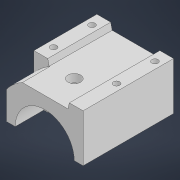
# Autodesk Inventor part: led_holder_01
Saved by Autodesk Inventor 2022 (Build 260153000, 153)
## iProperties
Created: 2025-10-28
Part Number: led_holder_01
Material: 一般
Document SubType Name: Modeling
Designer: gisen
Density: 1 g/cm^3
Appearance: 既定
Author: gisen
Autodesk Inventor part; units mm, degrees
ref_plane "YZ Plane" through (0, 0, 0) normal (1, 0, 0) x (0, 1, 0)
ref_plane "XZ Plane" through (0, 0, 0) normal (0, 1, 0) x (-1, 0, 0)
ref_plane "XY Plane" through (0, 0, 0) normal (0, 0, 1) x (1, 0, 0)
sketch "スケッチ1" plane through (0, 0, 0) normal (0, 0, 1) x (1, 0, 0)
  line L0 (-12.5, 3.2) -> (-11.75, 0)
  line L1 (-11.75, 0) -> (11.75, 0)
  line L2 (11.75, 0) -> (12.5, 3.2)
  line L3 (12.5, 3.2) -> (19.5, 3.2)
  line L4 (19.5, 3.2) -> (19.5, -4)
  line L5 (19.5, -4) -> (-19.5, -4)
  line L6 (-19.5, -4) -> (-19.5, 3.2)
  line L7 (-19.5, 3.2) -> (-12.5, 3.2)
  circle A0 centre (0, -21) radius 12.7 construction
  line L8 (-5.5, -4) -> (5.5, -4) construction
  line L9 (5.5, -4) -> (5.5, -7.5) construction
  line L10 (5.5, -7.5) -> (-5.5, -7.5) construction
  line L11 (-5.5, -7.5) -> (-5.5, -4) construction
  circle A1 centre (0, -21) radius 14.7 construction
  line L12 (-19.5, -21) -> (19.5, -21) construction
  line L13 (-18.75, -24.8) -> (-13.25, -24.8) construction
  line L14 (-13.25, -24.8) -> (-13.25, -27.8) construction
  line L15 (-13.25, -27.8) -> (-18.75, -27.8) construction
  line L16 (-18.75, -27.8) -> (-18.75, -24.8) construction
  line L17 (-16, -27.8) -> (-16, -14.8) construction
  line L18 (-18.75, -14.8) -> (-13.25, -14.8) construction
  line L19 (-13.25, -14.8) -> (-13.25, -17.2) construction
  line L20 (-13.25, -17.2) -> (-18.75, -17.2) construction
  line L21 (-18.75, -17.2) -> (-18.75, -14.8) construction
  line L22 (-14.5, -14.8) -> (-14.5, -27.8) construction
  line L23 (-17.5, -14.8) -> (-17.5, -27.8) construction
  point P0 (0, 0)
  point P1 (0, 0)
  point P2 (0, -4)
  dimension "d0" = 4
  dimension "d1" = 3.2
  dimension "d2" = 23.5
  dimension "d3" = 25
  dimension "d4" = 39
  dimension "d5" = 25.4
  dimension "d6" = 3.5
  dimension "d7" = 21
  dimension "d8" = 11
  dimension "d9" = 2
  dimension "d11" = 5.5
  dimension "d12" = 3
  dimension "d13" = 5.5
  dimension "d14" = 2.4
  dimension "d15" = 10
  dimension "d16" = 1.5
  dimension "d17" = 1.5
  dimension "d18" = 3.8
  dimension "d19" = 16
  constraints: 48 end point, 8 parallel, 8 perpendicular, 6 midpoint, 5 horizontal, 5 point on line, 3 equal length, 3 vertical alignment, 2 centre point, 2 coincident, 1 vertical
  measures "d0" distance between parallel lines of L5 L1
  measures "d1" distance between parallel lines of L1 L3
  measures "d2" distance of L0.end L1.end
  measures "d3" distance of L2.end L0.start
  measures "d4" distance between parallel lines of L4 L6
  measures "d5" diameter of A0
  measures "d6" distance of L8.end L9.end
  measures "d7" distance from line of A0.centre L1
  measures "d8" distance of L9.end L10.end
  measures "d9" radial gap between concentric circles of A1 A0
  measures "d11" distance of L13.start L13.end
  measures "d12" distance of L15.end L13.start
  measures "d13" distance of L18.start L18.end
  measures "d14" distance of L20.end L18.start
  measures "d15" distance between parallel lines of L13 L18
  measures "d16" distance between parallel lines of L22 L17
  measures "d17" distance between parallel lines of L17 L23
  measures "d18" distance between parallel lines of L13 L12
  measures "d19" distance from line of A1.centre L17
extrude "押し出し1" add sketch "スケッチ1" along normal blind 46
sketch "スケッチ2" plane through (0, 0, 0) normal (0, 0, -1) x (-1, 0, 0)
  line L0 (19.5, -4) -> (-19.5, -4) projected
  circle A0 centre (0, -21) radius 12.7 projected
  line L1 (19.5, -21) -> (-19.5, -21) projected
  line L2 (-19.5, -21) -> (-19.5, -4)
  line L3 (19.5, -4) -> (19.5, -21)
  point P0 (0, 0)
  point P1 (-12.7, -21)
  point P2 (12.7, -21)
  constraints: 4 end point, 1 parallel, 1 vertical
extrude "押し出し2" add sketch "スケッチ2" against normal blind 31.5 contours L3 L1 A0 L2 L0
sketch "スケッチ3" plane through (0, 0, 31.5) normal (0, 0, 1) x (1, 0, 0)
  line L0 (-19.5, -4) -> (19.5, -4) projected
  line L1 (-19.5, -4) -> (-19.5, -21) projected
  line L2 (-19.5, -21) -> (-12.7, -21) projected
  arc A0 (12.7, -21) -> (-12.7, -21) centre (0, -21) ccw projected
  line L3 (12.7, -21) -> (19.5, -21) projected
  line L4 (19.5, -21) -> (19.5, -4) projected
  circle A1 centre (0, -21) radius 15
  point P0 (0, 0)
  point P1 (-15, -21)
  point P2 (15, -21)
  dimension "d24" = 30
  constraints: 1 centre point, 1 coincident
  measures "d24" diameter of A1
extrude "押し出し3" add sketch "スケッチ3" along normal up to surface (14.5 mm away) contours L0 L4 L3 A1 L2 L1
sketch "スケッチ5" plane through (0, 0, 0) normal (0, 1, 0) x (-1, 0, 0)
  circle A0 centre (0, 31) radius 5.5
  line L0 (-11.75, 46) -> (11.75, 46) projected
  point P0 (0, 0)
  point P1 (0, 46)
  dimension "d27" = 15
  dimension "d28" = 11
  constraints: 1 centre point, 1 midpoint, 1 vertical alignment
  measures "d27" distance from line of A0.centre L0
  measures "d28" diameter of A0
extrude "押し出し4" cut sketch "スケッチ5" along normal through all both and the other way through all
sketch "スケッチ6" plane through (-11.75, 0, 0) normal (0, 1, 0) x (1, 0, 0)
  circle A0 centre (11.75, -31) radius 5.5 projected
  circle A1 centre (11.75, -31) radius 3.2
  point P0 (11.75, 0)
  dimension "d31" = 6.4
  constraints: 1 centre point, 1 coincident
  measures "d31" diameter of A1
extrude "押し出し5" add sketch "スケッチ6" against normal blind 4
sketch "スケッチ7" plane through (-19.5, -21, 0) normal (0, -1, 0) x (1, 0, 0)
  line L0 (6.8, 0) -> (0, 0) construction
  line L1 (6.8, 0) -> (6.8, 31.5) construction
  line L2 (4.5, 31.5) -> (6.8, 31.5) construction
  line L3 (4.5, 31.5) -> (4.5, 46) construction
  line L4 (4.5, 46) -> (0, 46) construction
  line L5 (0, 0) -> (0, 46) construction
  line L6 (3.5, 0) -> (3.5, 31.5) construction
  circle A0 centre (3.5, 6) radius 2.25
  circle A1 centre (3.5, 25.5) radius 2.25
  point P0 (19.5, 0)
  dimension "d34" = 16
  dimension "d35" = 4.5
  dimension "d36" = 6
  dimension "d37" = 6
  constraints: 3 point on line, 2 centre point, 2 end point, 1 equal radius, 1 vertical
  measures "d34" distance from line of L6 point (19.5, 0)
  measures "d35" diameter of A0
  measures "d36" distance from line of A0.centre L0
  measures "d37" distance from line of L2 A1.centre
extrude "押し出し6" cut sketch "スケッチ7" against normal blind 5
sketch "スケッチ8" plane through (-16, -16, 6) normal (0, -1, 0) x (1, 0, 0)
  circle A0 centre (0, 0) radius 2.25 projected
  circle A1 centre (0, 19.5) radius 2.25 projected
  circle A2 centre (0, 0) radius 1.6
  circle A3 centre (0, 19.5) radius 1.6
  point P0 (16, -6)
  dimension "d40" = 3.2
  constraints: 2 centre point, 2 coincident, 1 equal radius
  measures "d40" diameter of A2
extrude "押し出し7" cut sketch "スケッチ8" against normal through all contours A2 | A3
mirror "ミラー1" about plane through (0, 0, 0) normal (1, 0, 0) of "押し出し7", "押し出し6"
sketch "スケッチ9" plane through (-11.75, 0, 0) normal (0, 1, 0) x (1, 0, 0)
  line L0 (-7.75, -46) -> (3.9203, -46)
  line L1 (3.9203, -46) -> (3.9203, -32)
  line L2 (3.9203, -32) -> (-7.75, -32)
  line L3 (-7.75, -32) -> (-7.75, -46)
  point P0 (11.75, 0)
  dimension "d43" = 14
  constraints: 8 end point, 2 parallel, 1 horizontal, 1 perpendicular
  measures "d43" distance of L0.end L1.end
extrude "押し出し8" cut sketch "スケッチ9" along normal blind 10
sketch "スケッチ10" plane through (0, 0, 0) normal (1, 0, 0) x (0, 1, 0)
  line L0 (0, 0) -> (0, 46) projected
  line L1 (3.2, 46) -> (-21, 46) projected
  line L2 (3.2, 0) -> (-21, 0) projected
  line L3 (0, 0) -> (0.2, 46)
  dimension "d46" = 0.2
  constraints: 2 end point, 1 point on line
  measures "d46" distance from line of L0 L3.end
extrude "押し出し9" add sketch "スケッチ10" along normal up to surface surface through (12.5, 3.2, 0) normal (-0.9736163, 0.2281913, 0)
mirror "ミラー2" about plane through (0, 0, 0) normal (1, 0, 0) of "押し出し9"
sketch "スケッチ11" plane through (0, -4, 31) normal (0, -1, 0) x (1, 0, 0)
  circle A0 centre (0, 0) radius 3.2 projected
  point P0 (0, -31)
extrude "押し出し10" cut sketch "スケッチ11" against normal through all
sketch "スケッチ12" plane through (0, 0, 46) normal (0, 0, 1) x (1, 0, 0)
  arc A0 (15, -21) -> (-15, -21) centre (0, -21) ccw projected
  arc A1 (-11.3852, 0.2) -> (-19.5, -6.8999) centre (0, -21) ccw
  line L0 (-19.5, 0) -> (-19.5, -21) projected
  line L1 (-19.5, 0) -> (-19.5, 3.2) projected
  line L2 (-19.5, 3.2) -> (-12.5, 3.2) projected
  line L3 (-12.5, 3.2) -> (-11.7826, 0.1391) projected
  line L4 (11.7969, 0.2) -> (-11.7969, 0.2) projected
  point P0 (0, 0)
  point P1 (-11.75, 0)
  constraints: 3 point on circle, 2 point on line, 1 centre point, 1 coincident
extrude "押し出し11" cut sketch "スケッチ12" against normal up to surface (14 mm away)
equation "\"d17\" = d16"
equation "\"d32\" = d0"
equation "\"d34\" = d19"
